Autodesk Inventor part; units mm, degrees
(part 2 of 2)
sketch "Sketch5" plane through (0, 0, 0) normal (0, -1, 0) x (1, 0, 0)
  line L0 (-3.9998, 36.3944) -> (-3.9998, -39.0251) construction
  line L1 (-3.9998, -39.0251) -> (-16.6321, -39.0251) construction
  line L2 (-16.6321, -39.0251) -> (-16.6321, 36.3944) construction
  line L3 (-16.6321, 36.3944) -> (-3.9998, 36.3944) construction
  line L4 (-10.3717, 31.8861) -> (-10.3717, 36.1472)
  line L5 (-10.3717, 36.1472) -> (-9.6154, 36.1472)
  line L6 (-9.6154, 36.1472) -> (-4.9934, 32.8847)
  line L7 (-4.9934, 32.8847) -> (-4.9934, 35.9989)
  line L8 (-4.9934, 35.9989) -> (-4.2717, 35.9989)
  line L9 (-4.2717, 35.9989) -> (-4.2717, 31.9702)
  line L10 (-4.2717, 31.9702) -> (-5.0033, 31.9702)
  line L11 (-5.0033, 31.9702) -> (-9.65, 35.2673)
  line L12 (-9.65, 35.2673) -> (-9.65, 31.8861)
  line L13 (-9.65, 31.8861) -> (-10.3717, 31.8861)
  line L14 (-10.3717, 27.5509) -> (-10.3717, 28.322)
  line L15 (-10.3717, 28.322) -> (-7.7616, 28.322)
  spline S0 degree 2 poles (-7.7616, 28.322) (-7.4453, 28.322) (-6.9015, 28.3813) (-6.7384, 28.4703) knots 0 0 0 1 2 2 2
  spline S1 degree 2 poles (-6.7384, 28.4703) (-6.5654, 28.5643) (-6.3973, 28.9004) (-6.3973, 29.1871) knots 0 0 0 1 2 2 2
  spline S2 degree 2 poles (-6.3973, 29.1871) (-6.3973, 29.4738) (-6.7038, 30.0818) (-6.9509, 30.3735) knots 0 0 0 1 2 2 2
  line L16 (-6.9509, 30.3735) -> (-10.3717, 30.3735)
  line L17 (-10.3717, 30.3735) -> (-10.3717, 31.1446)
  line L18 (-10.3717, 31.1446) -> (-3.9998, 31.1446)
  line L19 (-3.9998, 31.1446) -> (-3.9998, 30.3735)
  line L20 (-3.9998, 30.3735) -> (-6.3034, 30.3735)
  spline S3 degree 2 poles (-6.3034, 30.3735) (-5.9919, 30.0275) (-5.6657, 29.3601) (-5.6657, 28.9844) knots 0 0 0 1 2 2 2
  spline S4 degree 2 poles (-5.6657, 28.9844) (-5.6657, 28.3121) (-6.5555, 27.5509) (-7.4008, 27.5509) knots 0 0 0 1 2 2 2
  line L21 (-7.4008, 27.5509) -> (-10.3717, 27.5509)
  line L22 (-10.3717, 25.6823) -> (-10.3717, 26.4535)
  line L23 (-10.3717, 26.4535) -> (-5.7942, 26.4535)
  line L24 (-5.7942, 26.4535) -> (-5.7942, 25.6823)
  line L25 (-5.7942, 25.6823) -> (-10.3717, 25.6823)
  line L26 (-5.0329, 25.6279) -> (-5.0329, 26.5029)
  line L27 (-5.0329, 26.5029) -> (-4.2321, 26.5029)
  line L28 (-4.2321, 26.5029) -> (-4.2321, 25.6279)
  line L29 (-4.2321, 25.6279) -> (-5.0329, 25.6279)
  line L30 (-10.3717, 23.0673) -> (-4.9934, 23.0673)
  line L31 (-4.9934, 23.0673) -> (-4.9934, 25.1138)
  line L32 (-4.9934, 25.1138) -> (-4.2717, 25.1138)
  line L33 (-4.2717, 25.1138) -> (-4.2717, 20.2101)
  line L34 (-4.2717, 20.2101) -> (-4.9934, 20.2101)
  line L35 (-4.9934, 20.2101) -> (-4.9934, 22.2566)
  line L36 (-4.9934, 22.2566) -> (-10.3717, 22.2566)
  line L37 (-10.3717, 22.2566) -> (-10.3717, 23.0673)
  spline S5 degree 2 poles (-10.4755, 17.6643) (-10.4755, 18.7617) (-9.2446, 19.9679) (-8.1077, 19.9679) knots 0 0 0 1 2 2 2
  spline S6 degree 2 poles (-8.1077, 19.9679) (-6.9905, 19.9679) (-5.6657, 18.7963) (-5.6657, 17.8522) knots 0 0 0 1 2 2 2
  spline S7 degree 2 poles (-5.6657, 17.8522) (-5.6657, 17.4271) (-5.9128, 16.7696) (-6.1748, 16.5274) knots 0 0 0 1 2 2 2
  spline S8 degree 2 poles (-6.1748, 16.5274) (-6.4368, 16.2802) (-7.1932, 16.0182) (-7.7419, 16.0182) knots 0 0 0 1 2 2 2
  line L38 (-7.7419, 16.0182) -> (-8.162, 16.0182)
  line L39 (-8.162, 16.0182) -> (-8.162, 19.1869)
  spline S9 degree 2 poles (-8.162, 19.1869) (-8.9579, 19.1869) (-9.8032, 18.386) (-9.8032, 17.6742) knots 0 0 0 1 2 2 2
  spline S10 degree 2 poles (-9.8032, 17.6742) (-9.8032, 17.4221) (-9.6895, 16.9327) (-9.6005, 16.735) knots 0 0 0 1 2 2 2
  spline S11 degree 2 poles (-9.6005, 16.735) (-9.5017, 16.5274) (-9.3286, 16.2407) (-9.2496, 16.1467) knots 0 0 0 1 2 2 2
  line L40 (-9.2496, 16.1467) -> (-9.2496, 16.1023)
  line L41 (-9.2496, 16.1023) -> (-10.0899, 16.1023)
  spline S12 degree 2 poles (-10.0899, 16.1023) (-10.1443, 16.2357) (-10.3025, 16.6411) (-10.347, 16.7993) knots 0 0 0 1 2 2 2
  spline S13 degree 2 poles (-10.347, 16.7993) (-10.4112, 17.0217) (-10.4755, 17.3875) (-10.4755, 17.6643) knots 0 0 0 1 2 2 2
  spline S14 degree 2 poles (-7.5738, 16.7696) (-7.2624, 16.7795) (-6.8076, 16.908) (-6.6543, 17.0316) knots 0 0 0 1 2 2 2
  spline S15 degree 2 poles (-6.6543, 17.0316) (-6.4813, 17.1651) (-6.2984, 17.5852) (-6.2984, 17.8967) knots 0 0 0 1 2 2 2
  spline S16 degree 2 poles (-6.2984, 17.8967) (-6.2984, 18.2031) (-6.4813, 18.6332) (-6.6593, 18.8112) knots 0 0 0 1 2 2 2
  spline S17 degree 2 poles (-6.6593, 18.8112) (-6.8422, 18.9842) (-7.2821, 19.1621) (-7.5738, 19.1869) knots 0 0 0 1 2 2 2
  line L42 (-7.5738, 19.1869) -> (-7.5738, 16.7696)
  spline S18 degree 2 poles (-10.4755, 13.4181) (-10.4755, 13.8926) (-10.1838, 14.6786) (-9.8872, 14.9604) knots 0 0 0 1 2 2 2
  spline S19 degree 2 poles (-9.8872, 14.9604) (-9.5956, 15.2421) (-8.6959, 15.5536) (-8.0928, 15.5536) knots 0 0 0 1 2 2 2
  spline S20 degree 2 poles (-8.0928, 15.5536) (-7.4897, 15.5536) (-6.6098, 15.2322) (-6.3133, 14.9604) knots 0 0 0 1 2 2 2
  spline S21 degree 2 poles (-6.3133, 14.9604) (-6.0117, 14.6885) (-5.6904, 13.8827) (-5.6904, 13.4181) knots 0 0 0 1 2 2 2
  spline S22 degree 2 poles (-5.6904, 13.4181) (-5.6904, 13.0424) (-5.903, 12.3404) (-6.0414, 12.0685) knots 0 0 0 1 2 2 2
  line L43 (-6.0414, 12.0685) -> (-6.9064, 12.0685)
  line L44 (-6.9064, 12.0685) -> (-6.9064, 12.113)
  spline S23 degree 2 poles (-6.9064, 12.113) (-6.8372, 12.1971) (-6.6593, 12.4541) (-6.5654, 12.637) knots 0 0 0 1 2 2 2
  spline S24 degree 2 poles (-6.5654, 12.637) (-6.4863, 12.8001) (-6.3627, 13.2352) (-6.3627, 13.4329) knots 0 0 0 1 2 2 2
  spline S25 degree 2 poles (-6.3627, 13.4329) (-6.3627, 14.031) (-7.2673, 14.7577) (-8.0928, 14.7577) knots 0 0 0 1 2 2 2
  spline S26 degree 2 poles (-8.0928, 14.7577) (-8.8986, 14.7577) (-9.8032, 14.0557) (-9.8032, 13.4329) knots 0 0 0 1 2 2 2
  spline S27 degree 2 poles (-9.8032, 13.4329) (-9.8032, 13.0572) (-9.4918, 12.375) (-9.2496, 12.113) knots 0 0 0 1 2 2 2
  line L45 (-9.2496, 12.113) -> (-9.2496, 12.0685)
  line L46 (-9.2496, 12.0685) -> (-10.1146, 12.0685)
  spline S28 degree 2 poles (-10.1146, 12.0685) (-10.169, 12.1822) (-10.3222, 12.5283) (-10.3568, 12.6667) knots 0 0 0 1 2 2 2
  spline S29 degree 2 poles (-10.3568, 12.6667) (-10.4162, 12.8644) (-10.4755, 13.1758) (-10.4755, 13.4181) knots 0 0 0 1 2 2 2
  line L47 (-10.3717, 7.7728) -> (-10.3717, 8.544)
  line L48 (-10.3717, 8.544) -> (-7.7616, 8.544)
  spline S30 degree 2 poles (-7.7616, 8.544) (-7.4453, 8.544) (-6.9015, 8.6033) (-6.7384, 8.6923) knots 0 0 0 1 2 2 2
  spline S31 degree 2 poles (-6.7384, 8.6923) (-6.5654, 8.7862) (-6.3973, 9.1224) (-6.3973, 9.4091) knots 0 0 0 1 2 2 2
  spline S32 degree 2 poles (-6.3973, 9.4091) (-6.3973, 9.6958) (-6.7038, 10.3038) (-6.9509, 10.5954) knots 0 0 0 1 2 2 2
  line L49 (-6.9509, 10.5954) -> (-10.3717, 10.5954)
  line L50 (-10.3717, 10.5954) -> (-10.3717, 11.3666)
  line L51 (-10.3717, 11.3666) -> (-3.9998, 11.3666)
  line L52 (-3.9998, 11.3666) -> (-3.9998, 10.5954)
  line L53 (-3.9998, 10.5954) -> (-6.3034, 10.5954)
  spline S33 degree 2 poles (-6.3034, 10.5954) (-5.9919, 10.2494) (-5.6657, 9.5821) (-5.6657, 9.2064) knots 0 0 0 1 2 2 2
  spline S34 degree 2 poles (-5.6657, 9.2064) (-5.6657, 8.5341) (-6.5555, 7.7728) (-7.4008, 7.7728) knots 0 0 0 1 2 2 2
  line L54 (-7.4008, 7.7728) -> (-10.3717, 7.7728)
  line L55 (-10.3717, 4.6685) -> (-4.2717, 2.6121)
  line L56 (-4.2717, 2.6121) -> (-4.2717, 1.6135)
  line L57 (-4.2717, 1.6135) -> (-10.3717, -0.4429)
  line L58 (-10.3717, -0.4429) -> (-10.3717, 0.4123)
  line L59 (-10.3717, 0.4123) -> (-8.6662, 0.966)
  line L60 (-8.6662, 0.966) -> (-8.6662, 3.2942)
  line L61 (-8.6662, 3.2942) -> (-10.3717, 3.8479)
  line L62 (-10.3717, 3.8479) -> (-10.3717, 4.6685)
  line L63 (-7.9742, 1.1884) -> (-5.1021, 2.1326)
  line L64 (-5.1021, 2.1326) -> (-7.9742, 3.0718)
  line L65 (-7.9742, 3.0718) -> (-7.9742, 1.1884)
  line L66 (-10.3717, -3.1469) -> (-10.3717, -0.784)
  line L67 (-10.3717, -0.784) -> (-9.7488, -0.784)
  line L68 (-9.7488, -0.784) -> (-9.7488, -1.5601)
  line L69 (-9.7488, -1.5601) -> (-4.8945, -1.5601)
  line L70 (-4.8945, -1.5601) -> (-4.8945, -0.784)
  line L71 (-4.8945, -0.784) -> (-4.2717, -0.784)
  line L72 (-4.2717, -0.784) -> (-4.2717, -3.1469)
  line L73 (-4.2717, -3.1469) -> (-4.8945, -3.1469)
  line L74 (-4.8945, -3.1469) -> (-4.8945, -2.3708)
  line L75 (-4.8945, -2.3708) -> (-9.7488, -2.3708)
  line L76 (-9.7488, -2.3708) -> (-9.7488, -3.1469)
  line L77 (-9.7488, -3.1469) -> (-10.3717, -3.1469)
  line L78 (-10.3717, -6.1128) -> (-4.2717, -8.1692)
  line L79 (-4.2717, -8.1692) -> (-4.2717, -9.1678)
  line L80 (-4.2717, -9.1678) -> (-10.3717, -11.2242)
  line L81 (-10.3717, -11.2242) -> (-10.3717, -10.369)
  line L82 (-10.3717, -10.369) -> (-8.6662, -9.8153)
  line L83 (-8.6662, -9.8153) -> (-8.6662, -7.487)
  line L84 (-8.6662, -7.487) -> (-10.3717, -6.9334)
  line L85 (-10.3717, -6.9334) -> (-10.3717, -6.1128)
  line L86 (-7.9742, -9.5929) -> (-5.1021, -8.6487)
  line L87 (-5.1021, -8.6487) -> (-7.9742, -7.7095)
  line L88 (-7.9742, -7.7095) -> (-7.9742, -9.5929)
  spline S35 degree 2 poles (-10.4804, -12.979) (-10.4804, -12.5193) (-10.2333, -11.7234) (-10.0949, -11.4614) knots 0 0 0 1 2 2 2
  line L89 (-10.0949, -11.4614) -> (-9.2298, -11.4614)
  line L90 (-9.2298, -11.4614) -> (-9.2298, -11.501)
  spline S36 degree 2 poles (-9.2298, -11.501) (-9.3089, -11.5999) (-9.4967, -11.8668) (-9.6005, -12.0892) knots 0 0 0 1 2 2 2
  spline S37 degree 2 poles (-9.6005, -12.0892) (-9.6944, -12.282) (-9.8329, -12.7566) (-9.8329, -13.0087) knots 0 0 0 1 2 2 2
  spline S38 degree 2 poles (-9.8329, -13.0087) (-9.8329, -13.1916) (-9.7488, -13.6118) (-9.6796, -13.7106) knots 0 0 0 1 2 2 2
  spline S39 degree 2 poles (-9.6796, -13.7106) (-9.5857, -13.854) (-9.3731, -13.9825) (-9.1556, -13.9825) knots 0 0 0 1 2 2 2
  spline S40 degree 2 poles (-9.1556, -13.9825) (-8.8838, -13.9825) (-8.602, -13.6859) (-8.5081, -13.3053) knots 0 0 0 1 2 2 2
  spline S41 degree 2 poles (-8.5081, -13.3053) (-8.4735, -13.157) (-8.3746, -12.6824) (-8.3202, -12.4798) knots 0 0 0 1 2 2 2
  spline S42 degree 2 poles (-8.3202, -12.4798) (-8.167, -11.9558) (-7.5342, -11.4812) (-7.0844, -11.4812) knots 0 0 0 1 2 2 2
  spline S43 degree 2 poles (-7.0844, -11.4812) (-6.4615, -11.4812) (-5.6855, -12.4155) (-5.6855, -13.1866) knots 0 0 0 1 2 2 2
  spline S44 degree 2 poles (-5.6855, -13.1866) (-5.6855, -13.5673) (-5.8733, -14.3384) (-6.0167, -14.6004) knots 0 0 0 1 2 2 2
  line L91 (-6.0167, -14.6004) -> (-6.8422, -14.6004)
  line L92 (-6.8422, -14.6004) -> (-6.8422, -14.5609)
  spline S45 degree 2 poles (-6.8422, -14.5609) (-6.6049, -14.2643) (-6.333, -13.5426) (-6.333, -13.1718) knots 0 0 0 1 2 2 2
  spline S46 degree 2 poles (-6.333, -13.1718) (-6.333, -12.7912) (-6.6543, -12.2672) (-6.9756, -12.2672) knots 0 0 0 1 2 2 2
  spline S47 degree 2 poles (-6.9756, -12.2672) (-7.2673, -12.2672) (-7.5491, -12.5786) (-7.638, -12.9246) knots 0 0 0 1 2 2 2
  spline S48 degree 2 poles (-7.638, -12.9246) (-7.6825, -13.0927) (-7.7715, -13.5178) (-7.8259, -13.7502) knots 0 0 0 1 2 2 2
  spline S49 degree 2 poles (-7.8259, -13.7502) (-7.9544, -14.2544) (-8.5427, -14.7685) (-9.0518, -14.7685) knots 0 0 0 1 2 2 2
  spline S50 degree 2 poles (-9.0518, -14.7685) (-9.3484, -14.7685) (-9.8724, -14.5362) (-10.0652, -14.3088) knots 0 0 0 1 2 2 2
  spline S51 degree 2 poles (-10.0652, -14.3088) (-10.2679, -14.0665) (-10.4804, -13.4486) (-10.4804, -12.979) knots 0 0 0 1 2 2 2
  spline S52 degree 2 poles (-10.4804, -16.7211) (-10.4804, -16.2614) (-10.2333, -15.4655) (-10.0949, -15.2035) knots 0 0 0 1 2 2 2
  line L93 (-10.0949, -15.2035) -> (-9.2298, -15.2035)
  line L94 (-9.2298, -15.2035) -> (-9.2298, -15.243)
  spline S53 degree 2 poles (-9.2298, -15.243) (-9.3089, -15.3419) (-9.4967, -15.6088) (-9.6005, -15.8313) knots 0 0 0 1 2 2 2
  spline S54 degree 2 poles (-9.6005, -15.8313) (-9.6944, -16.0241) (-9.8329, -16.4986) (-9.8329, -16.7507) knots 0 0 0 1 2 2 2
  spline S55 degree 2 poles (-9.8329, -16.7507) (-9.8329, -16.9336) (-9.7488, -17.3538) (-9.6796, -17.4527) knots 0 0 0 1 2 2 2
  spline S56 degree 2 poles (-9.6796, -17.4527) (-9.5857, -17.596) (-9.3731, -17.7246) (-9.1556, -17.7246) knots 0 0 0 1 2 2 2
  spline S57 degree 2 poles (-9.1556, -17.7246) (-8.8838, -17.7246) (-8.602, -17.428) (-8.5081, -17.0473) knots 0 0 0 1 2 2 2
  spline S58 degree 2 poles (-8.5081, -17.0473) (-8.4735, -16.899) (-8.3746, -16.4245) (-8.3202, -16.2218) knots 0 0 0 1 2 2 2
  spline S59 degree 2 poles (-8.3202, -16.2218) (-8.167, -15.6978) (-7.5342, -15.2233) (-7.0844, -15.2233) knots 0 0 0 1 2 2 2
  spline S60 degree 2 poles (-7.0844, -15.2233) (-6.4615, -15.2233) (-5.6855, -16.1575) (-5.6855, -16.9287) knots 0 0 0 1 2 2 2
  spline S61 degree 2 poles (-5.6855, -16.9287) (-5.6855, -17.3093) (-5.8733, -18.0805) (-6.0167, -18.3425) knots 0 0 0 1 2 2 2
  line L95 (-6.0167, -18.3425) -> (-6.8422, -18.3425)
  line L96 (-6.8422, -18.3425) -> (-6.8422, -18.3029)
  spline S62 degree 2 poles (-6.8422, -18.3029) (-6.6049, -18.0063) (-6.333, -17.2846) (-6.333, -16.9139) knots 0 0 0 1 2 2 2
  spline S63 degree 2 poles (-6.333, -16.9139) (-6.333, -16.5332) (-6.6543, -16.0093) (-6.9756, -16.0093) knots 0 0 0 1 2 2 2
  spline S64 degree 2 poles (-6.9756, -16.0093) (-7.2673, -16.0093) (-7.5491, -16.3207) (-7.638, -16.6667) knots 0 0 0 1 2 2 2
  spline S65 degree 2 poles (-7.638, -16.6667) (-7.6825, -16.8348) (-7.7715, -17.2599) (-7.8259, -17.4922) knots 0 0 0 1 2 2 2
  spline S66 degree 2 poles (-7.8259, -17.4922) (-7.9544, -17.9964) (-8.5427, -18.5105) (-9.0518, -18.5105) knots 0 0 0 1 2 2 2
  spline S67 degree 2 poles (-9.0518, -18.5105) (-9.3484, -18.5105) (-9.8724, -18.2782) (-10.0652, -18.0508) knots 0 0 0 1 2 2 2
  spline S68 degree 2 poles (-10.0652, -18.0508) (-10.2679, -17.8086) (-10.4804, -17.1907) (-10.4804, -16.7211) knots 0 0 0 1 2 2 2
  line L97 (-10.3717, -20.0133) -> (-10.3717, -19.2422)
  line L98 (-10.3717, -19.2422) -> (-5.7942, -19.2422)
  line L99 (-5.7942, -19.2422) -> (-5.7942, -20.0133)
  line L100 (-5.7942, -20.0133) -> (-10.3717, -20.0133)
  line L101 (-5.0329, -20.0677) -> (-5.0329, -19.1927)
  line L102 (-5.0329, -19.1927) -> (-4.2321, -19.1927)
  line L103 (-4.2321, -19.1927) -> (-4.2321, -20.0677)
  line L104 (-4.2321, -20.0677) -> (-5.0329, -20.0677)
  spline S69 degree 2 poles (-10.4804, -22.3811) (-10.4804, -21.9214) (-10.2333, -21.1255) (-10.0949, -20.8635) knots 0 0 0 1 2 2 2
  line L105 (-10.0949, -20.8635) -> (-9.2298, -20.8635)
  line L106 (-9.2298, -20.8635) -> (-9.2298, -20.9031)
  spline S70 degree 2 poles (-9.2298, -20.9031) (-9.3089, -21.002) (-9.4967, -21.2689) (-9.6005, -21.4913) knots 0 0 0 1 2 2 2
  spline S71 degree 2 poles (-9.6005, -21.4913) (-9.6944, -21.6841) (-9.8329, -22.1587) (-9.8329, -22.4108) knots 0 0 0 1 2 2 2
  spline S72 degree 2 poles (-9.8329, -22.4108) (-9.8329, -22.5937) (-9.7488, -23.0139) (-9.6796, -23.1127) knots 0 0 0 1 2 2 2
  spline S73 degree 2 poles (-9.6796, -23.1127) (-9.5857, -23.2561) (-9.3731, -23.3846) (-9.1556, -23.3846) knots 0 0 0 1 2 2 2
  spline S74 degree 2 poles (-9.1556, -23.3846) (-8.8838, -23.3846) (-8.602, -23.088) (-8.5081, -22.7074) knots 0 0 0 1 2 2 2
  spline S75 degree 2 poles (-8.5081, -22.7074) (-8.4735, -22.5591) (-8.3746, -22.0845) (-8.3202, -21.8819) knots 0 0 0 1 2 2 2
  spline S76 degree 2 poles (-8.3202, -21.8819) (-8.167, -21.3579) (-7.5342, -20.8833) (-7.0844, -20.8833) knots 0 0 0 1 2 2 2
  spline S77 degree 2 poles (-7.0844, -20.8833) (-6.4615, -20.8833) (-5.6855, -21.8176) (-5.6855, -22.5887) knots 0 0 0 1 2 2 2
  spline S78 degree 2 poles (-5.6855, -22.5887) (-5.6855, -22.9694) (-5.8733, -23.7405) (-6.0167, -24.0025) knots 0 0 0 1 2 2 2
  line L107 (-6.0167, -24.0025) -> (-6.8422, -24.0025)
  line L108 (-6.8422, -24.0025) -> (-6.8422, -23.963)
  spline S79 degree 2 poles (-6.8422, -23.963) (-6.6049, -23.6664) (-6.333, -22.9447) (-6.333, -22.5739) knots 0 0 0 1 2 2 2
  spline S80 degree 2 poles (-6.333, -22.5739) (-6.333, -22.1933) (-6.6543, -21.6693) (-6.9756, -21.6693) knots 0 0 0 1 2 2 2
  spline S81 degree 2 poles (-6.9756, -21.6693) (-7.2673, -21.6693) (-7.5491, -21.9807) (-7.638, -22.3268) knots 0 0 0 1 2 2 2
  spline S82 degree 2 poles (-7.638, -22.3268) (-7.6825, -22.4948) (-7.7715, -22.9199) (-7.8259, -23.1523) knots 0 0 0 1 2 2 2
  spline S83 degree 2 poles (-7.8259, -23.1523) (-7.9544, -23.6565) (-8.5427, -24.1706) (-9.0518, -24.1706) knots 0 0 0 1 2 2 2
  spline S84 degree 2 poles (-9.0518, -24.1706) (-9.3484, -24.1706) (-9.8724, -23.9383) (-10.0652, -23.7109) knots 0 0 0 1 2 2 2
  spline S85 degree 2 poles (-10.0652, -23.7109) (-10.2679, -23.4687) (-10.4804, -22.8507) (-10.4804, -22.3811) knots 0 0 0 1 2 2 2
  spline S86 degree 2 poles (-10.4607, -26.2715) (-10.4607, -25.6437) (-9.7439, -24.9368) (-8.9678, -24.9368) knots 0 0 0 1 2 2 2
  line L109 (-8.9678, -24.9368) -> (-6.4319, -24.9368)
  line L110 (-6.4319, -24.9368) -> (-6.4319, -24.4178)
  line L111 (-6.4319, -24.4178) -> (-5.7942, -24.4178)
  line L112 (-5.7942, -24.4178) -> (-5.7942, -24.9368)
  line L113 (-5.7942, -24.9368) -> (-4.4793, -24.9368)
  line L114 (-4.4793, -24.9368) -> (-4.4793, -25.708)
  line L115 (-4.4793, -25.708) -> (-5.7942, -25.708)
  line L116 (-5.7942, -25.708) -> (-5.7942, -27.1267)
  line L117 (-5.7942, -27.1267) -> (-6.4319, -27.1267)
  line L118 (-6.4319, -27.1267) -> (-6.4319, -25.708)
  line L119 (-6.4319, -25.708) -> (-8.6119, -25.708)
  spline S87 degree 2 poles (-8.6119, -25.708) (-8.9579, -25.708) (-9.3385, -25.7327) (-9.5017, -25.8167) knots 0 0 0 1 2 2 2
  spline S88 degree 2 poles (-9.5017, -25.8167) (-9.645, -25.8859) (-9.7884, -26.1973) (-9.7884, -26.4643) knots 0 0 0 1 2 2 2
  spline S89 degree 2 poles (-9.7884, -26.4643) (-9.7884, -26.6521) (-9.6747, -27.0031) (-9.6401, -27.0822) knots 0 0 0 1 2 2 2
  line L120 (-9.6401, -27.0822) -> (-9.6401, -27.1267)
  line L121 (-9.6401, -27.1267) -> (-10.3321, -27.1267)
  spline S90 degree 2 poles (-10.3321, -27.1267) (-10.3915, -26.9092) (-10.4607, -26.4643) (-10.4607, -26.2715) knots 0 0 0 1 2 2 2
  spline S91 degree 2 poles (-9.8872, -30.2459) (-9.9564, -30.152) (-10.2036, -29.8356) (-10.2778, -29.6873) knots 0 0 0 1 2 2 2
  spline S92 degree 2 poles (-10.2778, -29.6873) (-10.3865, -29.4846) (-10.5002, -29.104) (-10.5002, -28.758) knots 0 0 0 1 2 2 2
  spline S93 degree 2 poles (-10.5002, -28.758) (-10.5002, -28.4762) (-10.2876, -27.967) (-10.0949, -27.7742) knots 0 0 0 1 2 2 2
  spline S94 degree 2 poles (-10.0949, -27.7742) (-9.907, -27.5913) (-9.3534, -27.3689) (-9.0469, -27.3689) knots 0 0 0 1 2 2 2
  spline S95 degree 2 poles (-9.0469, -27.3689) (-8.5723, -27.3689) (-7.9, -27.7693) (-7.7073, -28.2043) knots 0 0 0 1 2 2 2
  spline S96 degree 2 poles (-7.7073, -28.2043) (-7.5293, -28.5899) (-7.3958, -29.6379) (-7.3612, -30.2459) knots 0 0 0 1 2 2 2
  line L122 (-7.3612, -30.2459) -> (-7.2129, -30.2459)
  spline S97 degree 2 poles (-7.2129, -30.2459) (-6.946, -30.2459) (-6.6148, -30.0828) (-6.5209, -29.9345) knots 0 0 0 1 2 2 2
  spline S98 degree 2 poles (-6.5209, -29.9345) (-6.4269, -29.7862) (-6.3676, -29.361) (-6.3676, -29.1336) knots 0 0 0 1 2 2 2
  spline S99 degree 2 poles (-6.3676, -29.1336) (-6.3676, -28.8667) (-6.5258, -28.145) (-6.6791, -27.7841) knots 0 0 0 1 2 2 2
  line L123 (-6.6791, -27.7841) -> (-6.6791, -27.7396)
  line L124 (-6.6791, -27.7396) -> (-5.8931, -27.7396)
  spline S100 degree 2 poles (-5.8931, -27.7396) (-5.8338, -27.9522) (-5.6855, -28.7481) (-5.6855, -29.1386) knots 0 0 0 1 2 2 2
  spline S101 degree 2 poles (-5.6855, -29.1386) (-5.6855, -29.6131) (-5.8338, -30.2607) (-6.0265, -30.5178) knots 0 0 0 1 2 2 2
  spline S102 degree 2 poles (-6.0265, -30.5178) (-6.2144, -30.7699) (-6.8125, -31.017) (-7.2426, -31.017) knots 0 0 0 1 2 2 2
  line L125 (-7.2426, -31.017) -> (-10.3717, -31.017)
  line L126 (-10.3717, -31.017) -> (-10.3717, -30.2459)
  line L127 (-10.3717, -30.2459) -> (-9.8872, -30.2459)
  line L128 (-9.2446, -30.2459) -> (-7.9742, -30.2459)
  spline S103 degree 2 poles (-7.9742, -30.2459) (-7.9989, -29.9691) (-8.0829, -29.1336) (-8.162, -28.8717) knots 0 0 0 1 2 2 2
  spline S104 degree 2 poles (-8.162, -28.8717) (-8.256, -28.5652) (-8.6465, -28.1648) (-8.9925, -28.1648) knots 0 0 0 1 2 2 2
  spline S105 degree 2 poles (-8.9925, -28.1648) (-9.388, -28.1648) (-9.7884, -28.6097) (-9.7884, -29.0348) knots 0 0 0 1 2 2 2
  spline S106 degree 2 poles (-9.7884, -29.0348) (-9.7884, -29.3956) (-9.4769, -29.9888) (-9.2446, -30.2459) knots 0 0 0 1 2 2 2
  line L129 (-10.3717, -35.6934) -> (-10.3717, -34.9222)
  line L130 (-10.3717, -34.9222) -> (-7.7616, -34.9222)
  spline S107 degree 2 poles (-7.7616, -34.9222) (-7.4453, -34.9222) (-6.9015, -34.8629) (-6.7384, -34.7739) knots 0 0 0 1 2 2 2
  spline S108 degree 2 poles (-6.7384, -34.7739) (-6.5654, -34.68) (-6.3973, -34.3439) (-6.3973, -34.0571) knots 0 0 0 1 2 2 2
  spline S109 degree 2 poles (-6.3973, -34.0571) (-6.3973, -33.7704) (-6.7038, -33.1624) (-6.9509, -32.8708) knots 0 0 0 1 2 2 2
  line L131 (-6.9509, -32.8708) -> (-10.3717, -32.8708)
  line L132 (-10.3717, -32.8708) -> (-10.3717, -32.0996)
  line L133 (-10.3717, -32.0996) -> (-5.7942, -32.0996)
  line L134 (-5.7942, -32.0996) -> (-5.7942, -32.8708)
  line L135 (-5.7942, -32.8708) -> (-6.3034, -32.8708)
  spline S110 degree 2 poles (-6.3034, -32.8708) (-5.9919, -33.2168) (-5.6657, -33.8841) (-5.6657, -34.2598) knots 0 0 0 1 2 2 2
  spline S111 degree 2 poles (-5.6657, -34.2598) (-5.6657, -34.9321) (-6.5555, -35.6934) (-7.4008, -35.6934) knots 0 0 0 1 2 2 2
  line L136 (-7.4008, -35.6934) -> (-10.3717, -35.6934)
  spline S112 degree 2 poles (-10.4607, -38.1601) (-10.4607, -37.5323) (-9.7439, -36.8254) (-8.9678, -36.8254) knots 0 0 0 1 2 2 2
  line L137 (-8.9678, -36.8254) -> (-6.4319, -36.8254)
  line L138 (-6.4319, -36.8254) -> (-6.4319, -36.3063)
  line L139 (-6.4319, -36.3063) -> (-5.7942, -36.3063)
  line L140 (-5.7942, -36.3063) -> (-5.7942, -36.8254)
  line L141 (-5.7942, -36.8254) -> (-4.4793, -36.8254)
  line L142 (-4.4793, -36.8254) -> (-4.4793, -37.5965)
  line L143 (-4.4793, -37.5965) -> (-5.7942, -37.5965)
  line L144 (-5.7942, -37.5965) -> (-5.7942, -39.0152)
  line L145 (-5.7942, -39.0152) -> (-6.4319, -39.0152)
  line L146 (-6.4319, -39.0152) -> (-6.4319, -37.5965)
  line L147 (-6.4319, -37.5965) -> (-8.6119, -37.5965)
  spline S113 degree 2 poles (-8.6119, -37.5965) (-8.9579, -37.5965) (-9.3385, -37.6212) (-9.5017, -37.7053) knots 0 0 0 1 2 2 2
  spline S114 degree 2 poles (-9.5017, -37.7053) (-9.645, -37.7745) (-9.7884, -38.0859) (-9.7884, -38.3529) knots 0 0 0 1 2 2 2
  spline S115 degree 2 poles (-9.7884, -38.3529) (-9.7884, -38.5407) (-9.6747, -38.8917) (-9.6401, -38.9708) knots 0 0 0 1 2 2 2
  line L148 (-9.6401, -38.9708) -> (-9.6401, -39.0152)
  line L149 (-9.6401, -39.0152) -> (-10.3321, -39.0152)
  spline S116 degree 2 poles (-10.3321, -39.0152) (-10.3915, -38.7977) (-10.4607, -38.3529) (-10.4607, -38.1601) knots 0 0 0 1 2 2 2
  line L150 (-14.2806, 14.4507) -> (-16.5679, 15.0312)
  line L151 (-16.5679, 15.0312) -> (-16.5679, 15.3869)
  line L152 (-16.5679, 15.3869) -> (-14.8043, 15.9451)
  line L153 (-14.8043, 15.9451) -> (-16.5679, 16.5009)
  line L154 (-16.5679, 16.5009) -> (-16.5679, 16.8541)
  line L155 (-16.5679, 16.8541) -> (-14.2806, 17.4395)
  line L156 (-14.2806, 17.4395) -> (-14.2806, 17.0393)
  line L157 (-14.2806, 17.0393) -> (-16.0516, 16.6342)
  line L158 (-16.0516, 16.6342) -> (-14.2806, 16.0933)
  line L159 (-14.2806, 16.0933) -> (-14.2806, 15.7747)
  line L160 (-14.2806, 15.7747) -> (-16.0516, 15.2189)
  line L161 (-16.0516, 15.2189) -> (-14.2806, 14.8385)
  line L162 (-14.2806, 14.8385) -> (-14.2806, 14.4507)
  line L163 (-14.2806, 11.341) -> (-16.5679, 11.9214)
  line L164 (-16.5679, 11.9214) -> (-16.5679, 12.2771)
  line L165 (-16.5679, 12.2771) -> (-14.8043, 12.8354)
  line L166 (-14.8043, 12.8354) -> (-16.5679, 13.3911)
  line L167 (-16.5679, 13.3911) -> (-16.5679, 13.7443)
  line L168 (-16.5679, 13.7443) -> (-14.2806, 14.3297)
  line L169 (-14.2806, 14.3297) -> (-14.2806, 13.9296)
  line L170 (-14.2806, 13.9296) -> (-16.0516, 13.5245)
  line L171 (-16.0516, 13.5245) -> (-14.2806, 12.9836)
  line L172 (-14.2806, 12.9836) -> (-14.2806, 12.6649)
  line L173 (-14.2806, 12.6649) -> (-16.0516, 12.1092)
  line L174 (-16.0516, 12.1092) -> (-14.2806, 11.7288)
  line L175 (-14.2806, 11.7288) -> (-14.2806, 11.341)
  line L176 (-14.2806, 8.2312) -> (-16.5679, 8.8117)
  line L177 (-16.5679, 8.8117) -> (-16.5679, 9.1674)
  line L178 (-16.5679, 9.1674) -> (-14.8043, 9.7256)
  line L179 (-14.8043, 9.7256) -> (-16.5679, 10.2814)
  line L180 (-16.5679, 10.2814) -> (-16.5679, 10.6346)
  line L181 (-16.5679, 10.6346) -> (-14.2806, 11.22)
  line L182 (-14.2806, 11.22) -> (-14.2806, 10.8198)
  line L183 (-14.2806, 10.8198) -> (-16.0516, 10.4147)
  line L184 (-16.0516, 10.4147) -> (-14.2806, 9.8738)
  line L185 (-14.2806, 9.8738) -> (-14.2806, 9.5552)
  line L186 (-14.2806, 9.5552) -> (-16.0516, 8.9994)
  line L187 (-16.0516, 8.9994) -> (-14.2806, 8.619)
  line L188 (-14.2806, 8.619) -> (-14.2806, 8.2312)
  line L189 (-16.5679, 7.2951) -> (-16.5679, 7.7842)
  line L190 (-16.5679, 7.7842) -> (-15.985, 7.7842)
  line L191 (-15.985, 7.7842) -> (-15.985, 7.2951)
  line L192 (-15.985, 7.2951) -> (-16.5679, 7.2951)
  line L193 (-16.5679, 4.6497) -> (-16.5679, 6.7789)
  line L194 (-16.5679, 6.7789) -> (-16.19, 6.7789)
  line L195 (-16.19, 6.7789) -> (-13.8805, 5.1487)
  line L196 (-13.8805, 5.1487) -> (-13.8805, 6.7048)
  line L197 (-13.8805, 6.7048) -> (-13.5199, 6.7048)
  line L198 (-13.5199, 6.7048) -> (-13.5199, 4.6917)
  line L199 (-13.5199, 4.6917) -> (-13.8854, 4.6917)
  line L200 (-13.8854, 4.6917) -> (-16.2073, 6.3392)
  line L201 (-16.2073, 6.3392) -> (-16.2073, 4.6497)
  line L202 (-16.2073, 4.6497) -> (-16.5679, 4.6497)
  line L203 (-16.5679, 2.4835) -> (-16.5679, 2.8688)
  line L204 (-16.5679, 2.8688) -> (-15.2637, 2.8688)
  spline S117 degree 2 poles (-15.2637, 2.8688) (-15.1056, 2.8688) (-14.8339, 2.8985) (-14.7524, 2.9429) knots 0 0 0 1 2 2 2
  spline S118 degree 2 poles (-14.7524, 2.9429) (-14.666, 2.9899) (-14.582, 3.1578) (-14.582, 3.3011) knots 0 0 0 1 2 2 2
  spline S119 degree 2 poles (-14.582, 3.3011) (-14.582, 3.4444) (-14.7351, 3.7482) (-14.8586, 3.8939) knots 0 0 0 1 2 2 2
  line L205 (-14.8586, 3.8939) -> (-16.5679, 3.8939)
  line L206 (-16.5679, 3.8939) -> (-16.5679, 4.2792)
  line L207 (-16.5679, 4.2792) -> (-13.384, 4.2792)
  line L208 (-13.384, 4.2792) -> (-13.384, 3.8939)
  line L209 (-13.384, 3.8939) -> (-14.5351, 3.8939)
  spline S120 degree 2 poles (-14.5351, 3.8939) (-14.3794, 3.721) (-14.2164, 3.3875) (-14.2164, 3.1998) knots 0 0 0 1 2 2 2
  spline S121 degree 2 poles (-14.2164, 3.1998) (-14.2164, 2.8639) (-14.661, 2.4835) (-15.0834, 2.4835) knots 0 0 0 1 2 2 2
  line L210 (-15.0834, 2.4835) -> (-16.5679, 2.4835)
  line L211 (-16.5679, 1.5498) -> (-16.5679, 1.9352)
  line L212 (-16.5679, 1.9352) -> (-14.2806, 1.9352)
  line L213 (-14.2806, 1.9352) -> (-14.2806, 1.5498)
  line L214 (-14.2806, 1.5498) -> (-16.5679, 1.5498)
  line L215 (-13.9003, 1.5227) -> (-13.9003, 1.9599)
  line L216 (-13.9003, 1.9599) -> (-13.5001, 1.9599)
  line L217 (-13.5001, 1.9599) -> (-13.5001, 1.5227)
  line L218 (-13.5001, 1.5227) -> (-13.9003, 1.5227)
  line L219 (-16.5679, 0.2432) -> (-13.8805, 0.2432)
  line L220 (-13.8805, 0.2432) -> (-13.8805, 1.2658)
  line L221 (-13.8805, 1.2658) -> (-13.5199, 1.2658)
  line L222 (-13.5199, 1.2658) -> (-13.5199, -1.1845)
  line L223 (-13.5199, -1.1845) -> (-13.8805, -1.1845)
  line L224 (-13.8805, -1.1845) -> (-13.8805, -0.1619)
  line L225 (-13.8805, -0.1619) -> (-16.5679, -0.1619)
  line L226 (-16.5679, -0.1619) -> (-16.5679, 0.2432)
  spline S122 degree 2 poles (-16.6198, -2.4565) (-16.6198, -1.9082) (-16.0047, -1.3055) (-15.4366, -1.3055) knots 0 0 0 1 2 2 2
  spline S123 degree 2 poles (-15.4366, -1.3055) (-14.8784, -1.3055) (-14.2164, -1.8909) (-14.2164, -2.3627) knots 0 0 0 1 2 2 2
  spline S124 degree 2 poles (-14.2164, -2.3627) (-14.2164, -2.5751) (-14.3399, -2.9036) (-14.4708, -3.0246) knots 0 0 0 1 2 2 2
  spline S125 degree 2 poles (-14.4708, -3.0246) (-14.6017, -3.1481) (-14.9797, -3.279) (-15.2538, -3.279) knots 0 0 0 1 2 2 2
  line L227 (-15.2538, -3.279) -> (-15.4638, -3.279)
  line L228 (-15.4638, -3.279) -> (-15.4638, -1.6958)
  spline S126 degree 2 poles (-15.4638, -1.6958) (-15.8615, -1.6958) (-16.2838, -2.0959) (-16.2838, -2.4516) knots 0 0 0 1 2 2 2
  spline S127 degree 2 poles (-16.2838, -2.4516) (-16.2838, -2.5775) (-16.227, -2.8221) (-16.1826, -2.9209) knots 0 0 0 1 2 2 2
  spline S128 degree 2 poles (-16.1826, -2.9209) (-16.1332, -3.0246) (-16.0467, -3.1679) (-16.0072, -3.2148) knots 0 0 0 1 2 2 2
  line L229 (-16.0072, -3.2148) -> (-16.0072, -3.237)
  line L230 (-16.0072, -3.237) -> (-16.4271, -3.237)
  spline S129 degree 2 poles (-16.4271, -3.237) (-16.4543, -3.1704) (-16.5333, -2.9678) (-16.5555, -2.8888) knots 0 0 0 1 2 2 2
  spline S130 degree 2 poles (-16.5555, -2.8888) (-16.5876, -2.7776) (-16.6198, -2.5948) (-16.6198, -2.4565) knots 0 0 0 1 2 2 2
  spline S131 degree 2 poles (-15.1699, -2.9036) (-15.0142, -2.8987) (-14.787, -2.8344) (-14.7104, -2.7727) knots 0 0 0 1 2 2 2
  spline S132 degree 2 poles (-14.7104, -2.7727) (-14.624, -2.706) (-14.5326, -2.496) (-14.5326, -2.3404) knots 0 0 0 1 2 2 2
  spline S133 degree 2 poles (-14.5326, -2.3404) (-14.5326, -2.1873) (-14.624, -1.9724) (-14.7129, -1.8835) knots 0 0 0 1 2 2 2
  spline S134 degree 2 poles (-14.7129, -1.8835) (-14.8043, -1.797) (-15.0241, -1.7081) (-15.1699, -1.6958) knots 0 0 0 1 2 2 2
  line L231 (-15.1699, -1.6958) -> (-15.1699, -2.9036)
  spline S135 degree 2 poles (-16.6198, -4.5783) (-16.6198, -4.3411) (-16.474, -3.9484) (-16.3258, -3.8076) knots 0 0 0 1 2 2 2
  spline S136 degree 2 poles (-16.3258, -3.8076) (-16.1801, -3.6668) (-15.7305, -3.5112) (-15.4292, -3.5112) knots 0 0 0 1 2 2 2
  spline S137 degree 2 poles (-15.4292, -3.5112) (-15.1279, -3.5112) (-14.6882, -3.6718) (-14.54, -3.8076) knots 0 0 0 1 2 2 2
  spline S138 degree 2 poles (-14.54, -3.8076) (-14.3893, -3.9435) (-14.2288, -4.3461) (-14.2288, -4.5783) knots 0 0 0 1 2 2 2
  spline S139 degree 2 poles (-14.2288, -4.5783) (-14.2288, -4.766) (-14.335, -5.1167) (-14.4041, -5.2526) knots 0 0 0 1 2 2 2
  line L232 (-14.4041, -5.2526) -> (-14.8364, -5.2526)
  line L233 (-14.8364, -5.2526) -> (-14.8364, -5.2303)
  spline S140 degree 2 poles (-14.8364, -5.2303) (-14.8018, -5.1884) (-14.7129, -5.0599) (-14.666, -4.9685) knots 0 0 0 1 2 2 2
  spline S141 degree 2 poles (-14.666, -4.9685) (-14.6264, -4.887) (-14.5647, -4.6697) (-14.5647, -4.5709) knots 0 0 0 1 2 2 2
  spline S142 degree 2 poles (-14.5647, -4.5709) (-14.5647, -4.272) (-15.0167, -3.9089) (-15.4292, -3.9089) knots 0 0 0 1 2 2 2
  spline S143 degree 2 poles (-15.4292, -3.9089) (-15.8318, -3.9089) (-16.2838, -4.2596) (-16.2838, -4.5709) knots 0 0 0 1 2 2 2
  spline S144 degree 2 poles (-16.2838, -4.5709) (-16.2838, -4.7586) (-16.1282, -5.0994) (-16.0072, -5.2303) knots 0 0 0 1 2 2 2
  line L234 (-16.0072, -5.2303) -> (-16.0072, -5.2526)
  line L235 (-16.0072, -5.2526) -> (-16.4394, -5.2526)
  spline S145 degree 2 poles (-16.4394, -5.2526) (-16.4666, -5.1958) (-16.5432, -5.0229) (-16.5605, -4.9537) knots 0 0 0 1 2 2 2
  spline S146 degree 2 poles (-16.5605, -4.9537) (-16.5901, -4.8549) (-16.6198, -4.6993) (-16.6198, -4.5783) knots 0 0 0 1 2 2 2
  line L236 (-16.5679, -7.399) -> (-16.5679, -7.0137)
  line L237 (-16.5679, -7.0137) -> (-15.2637, -7.0137)
  spline S147 degree 2 poles (-15.2637, -7.0137) (-15.1056, -7.0137) (-14.8339, -6.9841) (-14.7524, -6.9396) knots 0 0 0 1 2 2 2
  spline S148 degree 2 poles (-14.7524, -6.9396) (-14.666, -6.8927) (-14.582, -6.7247) (-14.582, -6.5814) knots 0 0 0 1 2 2 2
  spline S149 degree 2 poles (-14.582, -6.5814) (-14.582, -6.4382) (-14.7351, -6.1344) (-14.8586, -5.9886) knots 0 0 0 1 2 2 2
  line L238 (-14.8586, -5.9886) -> (-16.5679, -5.9886)
  line L239 (-16.5679, -5.9886) -> (-16.5679, -5.6033)
  line L240 (-16.5679, -5.6033) -> (-13.384, -5.6033)
  line L241 (-13.384, -5.6033) -> (-13.384, -5.9886)
  line L242 (-13.384, -5.9886) -> (-14.5351, -5.9886)
  spline S150 degree 2 poles (-14.5351, -5.9886) (-14.3794, -6.1615) (-14.2164, -6.495) (-14.2164, -6.6827) knots 0 0 0 1 2 2 2
  spline S151 degree 2 poles (-14.2164, -6.6827) (-14.2164, -7.0186) (-14.661, -7.399) (-15.0834, -7.399) knots 0 0 0 1 2 2 2
  line L243 (-15.0834, -7.399) -> (-16.5679, -7.399)
  line L244 (-16.5679, -7.6411) -> (-13.5199, -8.6686)
  line L245 (-13.5199, -8.6686) -> (-13.5199, -9.1676)
  line L246 (-13.5199, -9.1676) -> (-16.5679, -10.1951)
  line L247 (-16.5679, -10.1951) -> (-16.5679, -9.7678)
  line L248 (-16.5679, -9.7678) -> (-15.7157, -9.4911)
  line L249 (-15.7157, -9.4911) -> (-15.7157, -8.3277)
  line L250 (-15.7157, -8.3277) -> (-16.5679, -8.0511)
  line L251 (-16.5679, -8.0511) -> (-16.5679, -7.6411)
  line L252 (-15.3699, -9.38) -> (-13.9348, -8.9082)
  line L253 (-13.9348, -8.9082) -> (-15.3699, -8.4389)
  line L254 (-15.3699, -8.4389) -> (-15.3699, -9.38)
  line L255 (-16.5679, -10.8472) -> (-16.5679, -10.4618)
  line L256 (-16.5679, -10.4618) -> (-14.2806, -10.4618)
  line L257 (-14.2806, -10.4618) -> (-14.2806, -10.8472)
  line L258 (-14.2806, -10.8472) -> (-16.5679, -10.8472)
  line L259 (-13.9003, -10.8743) -> (-13.9003, -10.4371)
  line L260 (-13.9003, -10.4371) -> (-13.5001, -10.4371)
  line L261 (-13.5001, -10.4371) -> (-13.5001, -10.8743)
  line L262 (-13.5001, -10.8743) -> (-13.9003, -10.8743)
  line L263 (-16.5679, -12.0105) -> (-16.5679, -11.5215)
  line L264 (-16.5679, -11.5215) -> (-15.985, -11.5215)
  line L265 (-15.985, -11.5215) -> (-15.985, -12.0105)
  line L266 (-15.985, -12.0105) -> (-16.5679, -12.0105)
  spline S152 degree 2 poles (-16.6198, -13.5914) (-16.6198, -13.3542) (-16.474, -12.9615) (-16.3258, -12.8207) knots 0 0 0 1 2 2 2
  spline S153 degree 2 poles (-16.3258, -12.8207) (-16.1801, -12.6799) (-15.7305, -12.5243) (-15.4292, -12.5243) knots 0 0 0 1 2 2 2
  spline S154 degree 2 poles (-15.4292, -12.5243) (-15.1279, -12.5243) (-14.6882, -12.6849) (-14.54, -12.8207) knots 0 0 0 1 2 2 2
  spline S155 degree 2 poles (-14.54, -12.8207) (-14.3893, -12.9566) (-14.2288, -13.3592) (-14.2288, -13.5914) knots 0 0 0 1 2 2 2
  spline S156 degree 2 poles (-14.2288, -13.5914) (-14.2288, -13.7791) (-14.335, -14.1298) (-14.4041, -14.2657) knots 0 0 0 1 2 2 2
  line L267 (-14.4041, -14.2657) -> (-14.8364, -14.2657)
  line L268 (-14.8364, -14.2657) -> (-14.8364, -14.2434)
  spline S157 degree 2 poles (-14.8364, -14.2434) (-14.8018, -14.2014) (-14.7129, -14.073) (-14.666, -13.9816) knots 0 0 0 1 2 2 2
  spline S158 degree 2 poles (-14.666, -13.9816) (-14.6264, -13.9001) (-14.5647, -13.6827) (-14.5647, -13.5839) knots 0 0 0 1 2 2 2
  spline S159 degree 2 poles (-14.5647, -13.5839) (-14.5647, -13.2851) (-15.0167, -12.922) (-15.4292, -12.922) knots 0 0 0 1 2 2 2
  spline S160 degree 2 poles (-15.4292, -12.922) (-15.8318, -12.922) (-16.2838, -13.2727) (-16.2838, -13.5839) knots 0 0 0 1 2 2 2
  spline S161 degree 2 poles (-16.2838, -13.5839) (-16.2838, -13.7717) (-16.1282, -14.1125) (-16.0072, -14.2434) knots 0 0 0 1 2 2 2
  line L269 (-16.0072, -14.2434) -> (-16.0072, -14.2657)
  line L270 (-16.0072, -14.2657) -> (-16.4394, -14.2657)
  spline S162 degree 2 poles (-16.4394, -14.2657) (-16.4666, -14.2089) (-16.5432, -14.036) (-16.5605, -13.9668) knots 0 0 0 1 2 2 2
  spline S163 degree 2 poles (-16.5605, -13.9668) (-16.5901, -13.868) (-16.6198, -13.7124) (-16.6198, -13.5914) knots 0 0 0 1 2 2 2
  spline S164 degree 2 poles (-15.4243, -16.4961) (-16.0022, -16.4961) (-16.6321, -15.9403) (-16.6321, -15.476) knots 0 0 0 1 2 2 2
  spline S165 degree 2 poles (-16.6321, -15.476) (-16.6321, -14.9993) (-15.9825, -14.4534) (-15.4243, -14.4534) knots 0 0 0 1 2 2 2
  spline S166 degree 2 poles (-15.4243, -14.4534) (-14.8512, -14.4534) (-14.2164, -15.0165) (-14.2164, -15.476) knots 0 0 0 1 2 2 2
  spline S167 degree 2 poles (-14.2164, -15.476) (-14.2164, -15.9403) (-14.8487, -16.4961) (-15.4243, -16.4961) knots 0 0 0 1 2 2 2
  spline S168 degree 2 poles (-15.4243, -16.0984) (-14.9797, -16.0984) (-14.5474, -15.7748) (-14.5474, -15.476) knots 0 0 0 1 2 2 2
  spline S169 degree 2 poles (-14.5474, -15.476) (-14.5474, -15.1771) (-14.9797, -14.8511) (-15.4243, -14.8511) knots 0 0 0 1 2 2 2
  spline S170 degree 2 poles (-15.4243, -14.8511) (-15.8565, -14.8511) (-16.3011, -15.1771) (-16.3011, -15.476) knots 0 0 0 1 2 2 2
  spline S171 degree 2 poles (-16.3011, -15.476) (-16.3011, -15.7724) (-15.8639, -16.0984) (-15.4243, -16.0984) knots 0 0 0 1 2 2 2
  line L271 (-16.5679, -19.4848) -> (-15.244, -19.4848)
  spline S172 degree 2 poles (-15.244, -19.4848) (-15.0859, -19.4848) (-14.8166, -19.4601) (-14.7425, -19.4206) knots 0 0 0 1 2 2 2
  spline S173 degree 2 poles (-14.7425, -19.4206) (-14.661, -19.3811) (-14.582, -19.2304) (-14.582, -19.0995) knots 0 0 0 1 2 2 2
  spline S174 degree 2 poles (-14.582, -19.0995) (-14.582, -18.9809) (-14.7277, -18.7092) (-14.866, -18.566) knots 0 0 0 1 2 2 2
  spline S175 degree 2 poles (-14.866, -18.566) (-14.9006, -18.5684) (-14.9969, -18.5734) (-15.0612, -18.5734) knots 0 0 0 1 2 2 2
  line L272 (-15.0612, -18.5734) -> (-16.5679, -18.5734)
  line L273 (-16.5679, -18.5734) -> (-16.5679, -18.1881)
  line L274 (-16.5679, -18.1881) -> (-15.244, -18.1881)
  spline S176 degree 2 poles (-15.244, -18.1881) (-15.0859, -18.1881) (-14.8166, -18.1634) (-14.7425, -18.1238) knots 0 0 0 1 2 2 2
  spline S177 degree 2 poles (-14.7425, -18.1238) (-14.661, -18.0843) (-14.582, -17.9336) (-14.582, -17.8027) knots 0 0 0 1 2 2 2
  spline S178 degree 2 poles (-14.582, -17.8027) (-14.582, -17.6792) (-14.7376, -17.4051) (-14.8586, -17.2766) knots 0 0 0 1 2 2 2
  line L275 (-14.8586, -17.2766) -> (-16.5679, -17.2766)
  line L276 (-16.5679, -17.2766) -> (-16.5679, -16.8913)
  line L277 (-16.5679, -16.8913) -> (-14.2806, -16.8913)
  line L278 (-14.2806, -16.8913) -> (-14.2806, -17.2766)
  line L279 (-14.2806, -17.2766) -> (-14.5326, -17.2766)
  spline S179 degree 2 poles (-14.5326, -17.2766) (-14.3819, -17.4273) (-14.2164, -17.7237) (-14.2164, -17.9015) knots 0 0 0 1 2 2 2
  spline S180 degree 2 poles (-14.2164, -17.9015) (-14.2164, -18.1041) (-14.4017, -18.4178) (-14.6116, -18.4993) knots 0 0 0 1 2 2 2
  spline S181 degree 2 poles (-14.6116, -18.4993) (-14.4165, -18.6746) (-14.2164, -19.0056) (-14.2164, -19.1983) knots 0 0 0 1 2 2 2
  spline S182 degree 2 poles (-14.2164, -19.1983) (-14.2164, -19.3465) (-14.3078, -19.5885) (-14.4116, -19.6775) knots 0 0 0 1 2 2 2
  spline S183 degree 2 poles (-14.4116, -19.6775) (-14.5153, -19.7689) (-14.8265, -19.8701) (-15.0612, -19.8701) knots 0 0 0 1 2 2 2
  line L280 (-15.0612, -19.8701) -> (-16.5679, -19.8701)
  line L281 (-16.5679, -19.8701) -> (-16.5679, -19.4848)
  point P0 (0, 0)
  constraints: 2 other
extrude "Extrusion4" add sketch "Sketch5" along normal blind 0.5
sketch "Sketch6" plane through (0, 0, 0) normal (0, -1, 0) x (1, 0, 0)
  line L0 (-22.9068, 60.3499) -> (24.0932, 60.3499) projected
  line L1 (-22.9068, 60.3499) -> (-17.9068, 60.3499)
  line L2 (-22.9068, 60.3499) -> (-22.9068, 55.3499)
  line L3 (-22.9068, -58.6501) -> (-22.9068, 60.3499) projected
  line L4 (-22.9068, 55.3499) -> (-17.9068, 60.3499)
  line L5 (-17.9068, 60.3499) -> (-15.9068, 60.3499)
  line L6 (-15.9068, 60.3499) -> (-22.9068, 53.3499)
  line L7 (-22.9068, 53.3499) -> (-22.9068, 48.3499)
  line L8 (-22.9068, 48.3499) -> (-10.9068, 60.3499)
  line L9 (-10.9068, 60.3499) -> (-8.9068, 60.3499)
  line L10 (-8.9068, 60.3499) -> (-22.9068, 46.3499)
  line L11 (-8.9068, 60.3499) -> (-3.9068, 60.3499)
  line L12 (-22.9068, 60.3499) -> (24.0932, 60.3499) projected
  line L13 (-3.9068, 60.3499) -> (-22.9068, 41.3499)
  line L14 (-22.9068, 41.3499) -> (-22.9068, 39.3499)
  line L15 (-22.9068, 39.3499) -> (-1.9068, 60.3499)
  point P0 (0, 0)
  dimension "d20" = 5
  dimension "d21" = 5
  dimension "d22" = 2
  dimension "d23" = 5
  dimension "d24" = 2
  dimension "d27" = 5
  dimension "d28" = 2
  constraints: 26 end point, 12 point on line, 4 parallel
  measures "d20" distance of L0.start L1.end
  measures "d21" distance of L0.start L2.end
  measures "d22" distance of L1.end L5.end
  measures "d23" distance of L6.end L7.end
  measures "d24" distance of L8.end L9.end
  measures "d27" distance of L9.end L11.end
  measures "d28" distance of L13.end L14.end
extrude "Extrusion5" cut sketch "Sketch6" against normal blind 0.5 contours L0 L6 L3 L4 | L0 L10 L3 L8 | L0 L15 L3 L13
equation "\"BendRadius\" = Thickness"
equation "\"BendReliefWidth\" = Thickness"
equation "\"BendReliefDepth\" = 0.5 * Thickness"
equation "\"CornerReliefSize\" = 4 * Thickness"
equation "\"MinimumRemnant\" = 2 * Thickness"
equation "\"TransitionRadius\" = BendRadius"
equation "\"JacobiRadiusSize\" = BendRadius"
equation "\"GapSize\" = Thickness"
equation "\"Thickness\" = 0.5"
body "Solid1"
